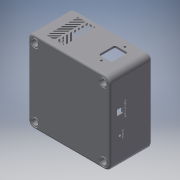
# Autodesk Inventor part: BottomBox
Saved by Autodesk Inventor 2019 (Build 230136000, 136)
## iProperties
Created: 2021-01-17
Part Number: BottomBox
Material: Типовые
Document SubType Name: Modeling
Designer: Dazer
Density: 1 g/cm^3
Appearance: По умолчанию
Author: Dazer
## iProperties of the stored document BottomBox_3DПЕЧАТЬ.ipt
Created: 2021-01-18
Part Number: BottomBox_3DПЕЧАТЬ
Material: Типовые
Document SubType Name: Modeling
Designer: Dazer
Density: 1 g/cm^3
Appearance: По умолчанию
Author: Dazer
Autodesk Inventor part; units mm, degrees
(part 1 of 2)
ref_plane "YZ Plane" through (0, 0, 0) normal (1, 0, 0) x (0, 1, 0)
ref_plane "XZ Plane" through (0, 0, 0) normal (0, 1, 0) x (-1, 0, 0)
ref_plane "XY Plane" through (0, 0, 0) normal (0, 0, 1) x (1, 0, 0)
sketch "Эскиз1" plane through (0, 0, 0) normal (0, 0, 1) x (1, 0, 0)
  circle A0 centre (1.5, -6.375) radius 2 projected
  circle A1 centre (88.9, -6.375) radius 2 projected
  circle A2 centre (88.9, -93.775) radius 2 projected
  circle A3 centre (1.5, -93.775) radius 2 projected
  arc A4 (87.4, -89.275) -> (84.4, -92.275) centre (87.4, -92.275) ccw projected
  line L0 (84.4, -92.275) -> (84.4, -96.775) projected
  arc A5 (81.4, -99.775) -> (84.4, -96.775) centre (81.4, -96.775) ccw projected
  line L1 (9, -99.775) -> (81.4, -99.775) projected
  arc A6 (6, -96.775) -> (9, -99.775) centre (9, -96.775) ccw projected
  line L2 (6, -96.775) -> (6, -92.275) projected
  arc A7 (6, -92.275) -> (3, -89.275) centre (3, -92.275) ccw projected
  line L3 (3, -89.275) -> (-1.5, -89.275) projected
  arc A8 (-4.5, -86.275) -> (-1.5, -89.275) centre (-1.5, -86.275) ccw projected
  line L4 (-4.5, -13.875) -> (-4.5, -86.275) projected
  arc A9 (-1.5, -10.875) -> (-4.5, -13.875) centre (-1.5, -13.875) ccw projected
  line L5 (-1.5, -10.875) -> (3, -10.875) projected
  arc A10 (3, -10.875) -> (6, -7.875) centre (3, -7.875) ccw projected
  line L6 (6, -7.875) -> (6, -3.375) projected
  arc A11 (9, -0.375) -> (6, -3.375) centre (9, -3.375) ccw projected
  line L7 (81.4, -0.375) -> (9, -0.375) projected
  arc A12 (84.4, -3.375) -> (81.4, -0.375) centre (81.4, -3.375) ccw projected
  line L8 (84.4, -3.375) -> (84.4, -7.875) projected
  arc A13 (84.4, -7.875) -> (87.4, -10.875) centre (87.4, -7.875) ccw projected
  line L9 (87.4, -10.875) -> (91.9, -10.875) projected
  arc A14 (94.9, -13.875) -> (91.9, -10.875) centre (91.9, -13.875) ccw projected
  line L10 (94.9, -86.275) -> (94.9, -13.875) projected
  arc A15 (91.9, -89.275) -> (94.9, -86.275) centre (91.9, -86.275) ccw projected
  line L11 (91.9, -89.275) -> (87.4, -89.275) projected
  line L12 (90.4, 0.875) -> (0, 0.875) projected
  arc A16 (0, 0.875) -> (-5.75, -4.875) centre (0, -4.875) ccw projected
  line L13 (-5.75, -4.875) -> (-5.75, -95.275) projected
  arc A17 (-5.75, -95.275) -> (0, -101.025) centre (0, -95.275) ccw projected
  line L14 (0, -101.025) -> (90.4, -101.025) projected
  arc A18 (90.4, -101.025) -> (96.15, -95.275) centre (90.4, -95.275) ccw projected
  line L15 (96.15, -95.275) -> (96.15, -4.875) projected
  arc A19 (96.15, -4.875) -> (90.4, 0.875) centre (90.4, -4.875) ccw projected
  line L16 (90.4, 0.775) -> (0, 0.775)
  arc A20 (0, 0.775) -> (-5.65, -4.875) centre (0, -4.875) ccw
  line L17 (-5.65, -4.875) -> (-5.65, -95.275)
  arc A21 (-5.65, -95.275) -> (0, -100.925) centre (0, -95.275) ccw
  line L18 (0, -100.925) -> (90.4, -100.925)
  arc A22 (90.4, -100.925) -> (96.05, -95.275) centre (90.4, -95.275) ccw
  line L19 (96.05, -95.275) -> (96.05, -4.875)
  arc A23 (96.05, -4.875) -> (90.4, 0.775) centre (90.4, -4.875) ccw
  circle A24 centre (88.9, -6.375) radius 2.3
  circle A25 centre (88.9, -93.775) radius 2.3
  circle A26 centre (1.5, -93.775) radius 2.3
  circle A27 centre (1.5, -6.375) radius 2.3
  point P0 (0, 0)
  dimension "d0" = 0.1
  dimension "d1" = 0.3
  dimension "d2" = 0.3
  dimension "d3" = 0.3
  dimension "d4" = 0.3
  constraints: 8 centre point, 8 end point, 8 point on circle, 7 other
  measures "d0" radial gap between concentric circles of A19 A23
  measures "d1" radial gap between concentric circles of A1 A24
  measures "d2" radial gap between concentric circles of A2 A25
  measures "d3" radial gap between concentric circles of A3 A26
  measures "d4" radial gap between concentric circles of A0 A27
extrude "Выдавливание1" add sketch "Эскиз1" along normal blind 2.1 contours A23 L19 A22 L18 A21 L17 A20 L16
sketch "Эскиз2" plane through (0, 0, 2.1) normal (0, 0, 1) x (1, 0, 0)
  arc A0 (96.15, -4.875) -> (90.4, 0.875) centre (90.4, -4.875) ccw projected
  line L0 (96.15, -4.875) -> (96.15, -95.275) projected
  arc A1 (90.4, -101.025) -> (96.15, -95.275) centre (90.4, -95.275) ccw projected
  line L1 (90.4, -101.025) -> (0, -101.025) projected
  arc A2 (-5.75, -95.275) -> (0, -101.025) centre (0, -95.275) ccw projected
  line L2 (-5.75, -95.275) -> (-5.75, -4.875) projected
  arc A3 (0, 0.875) -> (-5.75, -4.875) centre (0, -4.875) ccw projected
  line L3 (0, 0.875) -> (90.4, 0.875) projected
  line L4 (97.4, -95.275) -> (97.4, -4.875) projected
  arc A4 (97.4, -4.875) -> (90.4, 2.125) centre (90.4, -4.875) ccw projected
  line L5 (90.4, 2.125) -> (0, 2.125) projected
  arc A5 (0, 2.125) -> (-7, -4.875) centre (0, -4.875) ccw projected
  line L6 (-7, -4.875) -> (-7, -95.275) projected
  arc A6 (-7, -95.275) -> (0, -102.275) centre (0, -95.275) ccw projected
  line L7 (0, -102.275) -> (90.4, -102.275) projected
  arc A7 (90.4, -102.275) -> (97.4, -95.275) centre (90.4, -95.275) ccw projected
  line L8 (84.4, -92.275) -> (84.4, -96.775) projected
  arc A8 (81.4, -99.775) -> (84.4, -96.775) centre (81.4, -96.775) ccw projected
  line L9 (81.4, -99.775) -> (9, -99.775) projected
  arc A9 (6, -96.775) -> (9, -99.775) centre (9, -96.775) ccw projected
  line L10 (6, -96.775) -> (6, -92.275) projected
  arc A10 (6, -92.275) -> (3, -89.275) centre (3, -92.275) ccw projected
  line L11 (3, -89.275) -> (-1.5, -89.275) projected
  arc A11 (-4.5, -86.275) -> (-1.5, -89.275) centre (-1.5, -86.275) ccw projected
  line L12 (-4.5, -86.275) -> (-4.5, -13.875) projected
  arc A12 (-1.5, -10.875) -> (-4.5, -13.875) centre (-1.5, -13.875) ccw projected
  line L13 (-1.5, -10.875) -> (3, -10.875) projected
  arc A13 (3, -10.875) -> (6, -7.875) centre (3, -7.875) ccw projected
  line L14 (6, -7.875) -> (6, -3.375) projected
  arc A14 (9, -0.375) -> (6, -3.375) centre (9, -3.375) ccw projected
  line L15 (9, -0.375) -> (81.4, -0.375) projected
  arc A15 (84.4, -3.375) -> (81.4, -0.375) centre (81.4, -3.375) ccw projected
  line L16 (84.4, -3.375) -> (84.4, -7.875) projected
  arc A16 (84.4, -7.875) -> (87.4, -10.875) centre (87.4, -7.875) ccw projected
  line L17 (87.4, -10.875) -> (91.9, -10.875) projected
  arc A17 (94.9, -13.875) -> (91.9, -10.875) centre (91.9, -13.875) ccw projected
  line L18 (94.9, -13.875) -> (94.9, -86.275) projected
  arc A18 (91.9, -89.275) -> (94.9, -86.275) centre (91.9, -86.275) ccw projected
  line L19 (91.9, -89.275) -> (87.4, -89.275) projected
  arc A19 (87.4, -89.275) -> (84.4, -92.275) centre (87.4, -92.275) ccw projected
  circle A20 centre (1.5, -6.375) radius 2.3 projected
  circle A21 centre (1.5, -93.775) radius 2.3 projected
  circle A22 centre (88.9, -93.775) radius 2.3 projected
  circle A23 centre (88.9, -6.375) radius 2.3 projected
  line L20 (90.4, 0.775) -> (0, 0.775) projected
  arc A24 (0, 0.775) -> (-5.65, -4.875) centre (0, -4.875) ccw projected
  line L21 (-5.65, -4.875) -> (-5.65, -95.275) projected
  arc A25 (-5.65, -95.275) -> (0, -100.925) centre (0, -95.275) ccw projected
  line L22 (0, -100.925) -> (90.4, -100.925) projected
  arc A26 (90.4, -100.925) -> (96.05, -95.275) centre (90.4, -95.275) ccw projected
  line L23 (96.05, -95.275) -> (96.05, -4.875) projected
  arc A27 (96.05, -4.875) -> (90.4, 0.775) centre (90.4, -4.875) ccw projected
  point P0 (0, 0)
extrude "Выдавливание2" add sketch "Эскиз2" along normal blind 49 contours L0 A1 L1 A2 L2 A3 L3 A0 | A7 L7 A6 L6 A5 L5 A4 L4 | A27 L23 A26 L22 A25 L21 A24 L20
sketch "Эскиз3" plane through (0, 0, 51.1) normal (0, 0, 1) x (1, 0, 0)
  arc A0 (81.4, -99.775) -> (84.4, -96.775) centre (81.4, -96.775) ccw projected
  line L0 (81.4, -99.775) -> (9, -99.775) projected
  arc A1 (6, -96.775) -> (9, -99.775) centre (9, -96.775) ccw projected
  line L1 (6, -96.775) -> (6, -92.275) projected
  arc A2 (6, -92.275) -> (3, -89.275) centre (3, -92.275) ccw projected
  line L2 (3, -89.275) -> (-1.5, -89.275) projected
  arc A3 (-4.5, -86.275) -> (-1.5, -89.275) centre (-1.5, -86.275) ccw projected
  line L3 (-4.5, -86.275) -> (-4.5, -13.875) projected
  arc A4 (-1.5, -10.875) -> (-4.5, -13.875) centre (-1.5, -13.875) ccw projected
  line L4 (-1.5, -10.875) -> (3, -10.875) projected
  arc A5 (3, -10.875) -> (6, -7.875) centre (3, -7.875) ccw projected
  line L5 (6, -7.875) -> (6, -3.375) projected
  arc A6 (9, -0.375) -> (6, -3.375) centre (9, -3.375) ccw projected
  line L6 (9, -0.375) -> (81.4, -0.375) projected
  arc A7 (84.4, -3.375) -> (81.4, -0.375) centre (81.4, -3.375) ccw projected
  line L7 (84.4, -3.375) -> (84.4, -7.875) projected
  arc A8 (84.4, -7.875) -> (87.4, -10.875) centre (87.4, -7.875) ccw projected
  line L8 (87.4, -10.875) -> (91.9, -10.875) projected
  arc A9 (94.9, -13.875) -> (91.9, -10.875) centre (91.9, -13.875) ccw projected
  line L9 (94.9, -13.875) -> (94.9, -86.275) projected
  arc A10 (91.9, -89.275) -> (94.9, -86.275) centre (91.9, -86.275) ccw projected
  line L10 (91.9, -89.275) -> (87.4, -89.275) projected
  arc A11 (87.4, -89.275) -> (84.4, -92.275) centre (87.4, -92.275) ccw projected
  line L11 (84.4, -92.275) -> (84.4, -96.775) projected
  circle A12 centre (88.9, -6.375) radius 2.3 projected
  circle A13 centre (88.9, -93.775) radius 2.3 projected
  circle A14 centre (1.5, -93.775) radius 2.3 projected
  circle A15 centre (1.5, -6.375) radius 2.3 projected
  line L12 (97.4, -95.275) -> (97.4, -4.875) projected
  arc A16 (97.4, -4.875) -> (90.4, 2.125) centre (90.4, -4.875) ccw projected
  line L13 (90.4, 2.125) -> (0, 2.125) projected
  arc A17 (0, 2.125) -> (-7, -4.875) centre (0, -4.875) ccw projected
  line L14 (-7, -4.875) -> (-7, -95.275) projected
  arc A18 (-7, -95.275) -> (0, -102.275) centre (0, -95.275) ccw projected
  line L15 (0, -102.275) -> (90.4, -102.275) projected
  arc A19 (90.4, -102.275) -> (97.4, -95.275) centre (90.4, -95.275) ccw projected
  point P0 (0, 0)
extrude "Выдавливание3" add sketch "Эскиз3" along normal blind 2.5 contours L0 A1 L1 A2 L2 A3 L3 A4 L4 A5 L5 A6 L6 A7 L7 A8 L8 A9 L9 A10 L10 A11 L11 A0 | A19 L15 A18 L14 A17 L13 A16 L12
fillet "Сопряжение1" radius 2.5 8 edges at (-4.9497, -100.2247, 53.6) (45.2, -102.275, 53.6) (95.3497, -100.2247, 53.6) (97.4, -50.075, 53.6) (95.3497, 0.0747, 53.6) (45.2, 2.125, 53.6) (-4.9497, 0.0747, 53.6) (-7, -50.075, 53.6)
sketch "Эскиз5" plane through (0, 0, 53.6) normal (0, 0, 1) x (1, 0, 0)
  circle A0 centre (1.5, -6.375) radius 2.3 projected
  circle A1 centre (88.9, -6.375) radius 2.3 projected
  circle A2 centre (88.9, -93.775) radius 2.3 projected
  circle A3 centre (1.5, -93.775) radius 2.3 projected
  circle A4 centre (1.5, -93.775) radius 3.5
  circle A5 centre (88.9, -93.775) radius 3.5
  circle A6 centre (88.9, -6.375) radius 3.5
  circle A7 centre (1.5, -6.375) radius 3.5
  point P0 (0, 0)
  dimension "d22" = 7
  dimension "d23" = 7
  dimension "d24" = 7
  dimension "d25" = 7
  constraints: 4 centre point, 4 coincident
  measures "d22" diameter of A4
  measures "d23" diameter of A5
  measures "d24" diameter of A6
  measures "d25" diameter of A7
extrude "Выдавливание5" cut sketch "Эскиз5" against normal blind 39 contours A0 | A1 | A2 | A3 | A4 | A5 | A6 | A7
sketch "Эскиз6" plane through (97.4, -95.275, 2.1) normal (1, 0, 0) x (0, 0, -1)
  line L0 (-42.4, 54.65) -> (-42.4, 51.15)
  line L1 (-42.4, 58.15) -> (-42.4, 54.65)
  line L2 (-42.4, 58.15) -> (-34.78, 58.15)
  line L3 (-34.78, 58.15) -> (-34.78, 51.15)
  line L4 (-34.78, 51.15) -> (-42.4, 51.15)
  circle A0 centre (-38.59, 27.98) radius 1.5
  point P0 (2.1, 95.275)
  constraints: 10 end point, 1 centre point, 1 horizontal, 1 perpendicular, 1 point on line
extrude "Выдавливание6" cut sketch "Эскиз6" against normal blind 2.5
sketch "Эскиз7" plane through (0, 0, 51.1) normal (0, 0, -1) x (-1, 0, 0)
  arc A0 (-6, -7.875) -> (-3, -10.875) centre (-3, -7.875) ccw projected
  line L0 (-3, -89.275) -> (1.5, -89.275) projected
  line L1 (-3, -10.875) -> (-3, -89.275)
  line L2 (-3, -10.875) -> (1.5, -10.875)
  arc A1 (4.5, -13.875) -> (1.5, -10.875) centre (1.5, -13.875) ccw projected
  line L3 (4.5, -13.875) -> (4.5, -86.275)
  arc A2 (1.5, -89.275) -> (4.5, -86.275) centre (1.5, -86.275) ccw projected
  line L4 (-3, -89.275) -> (1.5, -89.275)
  arc A3 (1.5, -89.275) -> (4.5, -86.275) centre (1.5, -86.275) ccw
  arc A4 (4.5, -13.875) -> (1.5, -10.875) centre (1.5, -13.875) ccw
  point P0 (0, 0)
  constraints: 8 end point, 6 point on circle, 2 centre point, 2 tangent, 1 collinear, 1 concentric, 1 horizontal, 1 perpendicular, 1 vertical
extrude "Выдавливание7" add sketch "Эскиз7" along normal blind 5
sketch "Эскиз8" plane through (0, 0, 51.1) normal (0, 0, -1) x (-1, 0, 0)
  arc A0 (-6, -7.875) -> (-3, -10.875) centre (-3, -7.875) ccw projected
  line L0 (-6, -7.875) -> (-34, -7.875)
  line L1 (-34, -7.875) -> (-34, -0.375)
  line L2 (-34, -0.375) -> (-9, -0.375)
  arc A1 (-6, -3.375) -> (-9, -0.375) centre (-9, -3.375) ccw projected
  line L3 (-6, -3.375) -> (-6, -7.875)
  arc A2 (-6, -3.375) -> (-9, -0.375) centre (-9, -3.375) ccw
  line L4 (-6, -92.275) -> (-6, -96.775) projected
  line L5 (-6, -92.275) -> (-34, -92.275)
  line L6 (-34, -92.275) -> (-34, -99.775)
  line L7 (-81.4, -99.775) -> (-9, -99.775) projected
  arc A3 (-9, -99.775) -> (-6, -96.775) centre (-9, -96.775) ccw projected
  line L8 (-34, -99.775) -> (-9, -99.775)
  arc A4 (-3, -89.275) -> (-6, -92.275) centre (-3, -92.275) ccw projected
  line L9 (-6, -92.275) -> (-6, -96.775)
  arc A5 (-9, -99.775) -> (-6, -96.775) centre (-9, -96.775) ccw
  arc A6 (-84.4, -92.275) -> (-87.4, -89.275) centre (-87.4, -92.275) ccw projected
  line L10 (-84.4, -92.275) -> (-74.4, -92.275)
  line L11 (-74.4, -92.275) -> (-74.4, -99.775)
  line L12 (-9, -99.775) -> (-81.4, -99.775) projected
  line L13 (-74.4, -99.775) -> (-81.4, -99.775)
  arc A7 (-84.4, -96.775) -> (-81.4, -99.775) centre (-81.4, -96.775) ccw projected
  line L14 (-84.4, -92.275) -> (-84.4, -96.775)
  arc A8 (-84.4, -96.775) -> (-81.4, -99.775) centre (-81.4, -96.775) ccw
  line L15 (-64.4, -0.375) -> (-64.4, -7.375)
  line L16 (-64.4, -7.375) -> (-69.4, -7.375)
  line L17 (-69.4, -7.375) -> (-69.4, -0.375)
  line L18 (-69.4, -0.375) -> (-64.4, -0.375)
  point P0 (0, 0)
  dimension "d43" = 28
  dimension "d46" = 28
  dimension "d47" = 10
  constraints: 32 end point, 8 point on circle, 7 tangent, 6 horizontal, 4 perpendicular, 4 vertical, 3 centre point, 2 point on line, 1 concentric
  measures "d43" distance of L0.start L0.end
  measures "d46" distance of L4.start L5.end
  measures "d47" distance of L10.start L10.end
extrude "Выдавливание8" add sketch "Эскиз8" along normal blind 5
fillet "Сопряжение2" radius 2.5 5 edges at (34, -7.875, 48.6) (34, -92.275, 48.6) (74.4, -92.275, 48.6) (64.4, -7.375, 48.6) (69.4, -7.375, 48.6)
fillet "Сопряжение3" radius 2.5 12 edges at (49.2, -0.375, 51.1) (85.2787, -9.9963, 51.1) (89.65, -10.875, 51.1) (94.0213, -11.7537, 51.1) (94.9, -50.075, 51.1) (94.0213, -88.3963, 51.1) (89.65, -89.275, 51.1) (85.2787, -90.1537, 51.1) (83.5213, -1.2537, 51.1) (75.4, -0.375, 51.1) (84.4, -5.625, 51.1) (54.2, -99.775, 51.1)
fillet "Сопряжение4" radius 2.5 2 edges at (5.1213, -90.1537, 51.1) (5.1213, -9.9963, 51.1)
sketch "Эскиз9" plane through (0, 2.125, 2.1) normal (0, 1, 0) x (1, 0, 0)
  line L0 (9, -4) -> (11.5, -4)
  line L1 (9, -4) -> (9, -6.5)
  line L2 (9, -6.5) -> (11.5, -4)
  line L3 (9, -14) -> (19, -4)
  line L4 (9, -14) -> (9, -16.5)
  line L5 (9, -19) -> (9, -21.5)
  line L6 (9, -34) -> (9, -36.5)
  line L7 (9, -39) -> (9, -41.5)
  line L8 (19, -4) -> (19, -6.5)
  line L9 (19, -9) -> (19, -11.5)
  line L10 (19, -24) -> (19, -26.5)
  line L11 (19, -29) -> (19, -31.5)
  line L12 (9, -16.5) -> (19, -6.5)
  line L13 (9, -19) -> (19, -9)
  line L14 (9, -21.5) -> (19, -11.5)
  line L15 (9, -24) -> (19, -14)
  line L16 (9, -26.5) -> (19, -16.5)
  line L17 (9, -29) -> (19, -19)
  line L18 (9, -31.5) -> (19, -21.5)
  line L19 (9, -34) -> (19, -24)
  line L20 (9, -36.5) -> (19, -26.5)
  line L21 (9, -39) -> (19, -29)
  line L22 (9, -41.5) -> (19, -31.5)
  line L23 (9, -44) -> (19, -34)
  line L24 (11.5, -44) -> (19, -36.5)
  line L25 (14, -44) -> (19, -39)
  line L26 (16.5, -44) -> (19, -41.5)
  line L27 (9, -9) -> (14, -4)
  line L28 (9, -11.5) -> (16.5, -4)
  line L29 (14, -4) -> (16.5, -4)
  line L30 (9, -9) -> (9, -11.5)
  line L31 (19, -34) -> (19, -36.5)
  line L32 (11.5, -44) -> (9, -44)
  line L33 (14, -44) -> (16.5, -44)
  line L34 (19, -39) -> (19, -41.5)
  line L35 (9, -24) -> (9, -26.5)
  line L36 (19, -14) -> (19, -16.5)
  line L37 (9, -29) -> (9, -31.5)
  line L38 (19, -21.5) -> (19, -19)
  line L39 (31.5, -4) -> (29, -4)
  line L40 (31.5, -4) -> (31.5, -6.5)
  line L41 (31.5, -6.5) -> (29, -4)
  line L42 (31.5, -14) -> (21.5, -4)
  line L43 (31.5, -14) -> (31.5, -16.5)
  line L44 (31.5, -19) -> (31.5, -21.5)
  line L45 (31.5, -34) -> (31.5, -36.5)
  line L46 (31.5, -39) -> (31.5, -41.5)
  line L47 (21.5, -4) -> (21.5, -6.5)
  line L48 (21.5, -9) -> (21.5, -11.5)
  line L49 (21.5, -24) -> (21.5, -26.5)
  line L50 (21.5, -29) -> (21.5, -31.5)
  line L51 (31.5, -16.5) -> (21.5, -6.5)
  line L52 (31.5, -19) -> (21.5, -9)
  line L53 (31.5, -21.5) -> (21.5, -11.5)
  line L54 (31.5, -24) -> (21.5, -14)
  line L55 (31.5, -26.5) -> (21.5, -16.5)
  line L56 (31.5, -29) -> (21.5, -19)
  line L57 (31.5, -31.5) -> (21.5, -21.5)
  line L58 (31.5, -34) -> (21.5, -24)
  line L59 (31.5, -36.5) -> (21.5, -26.5)
  line L60 (31.5, -39) -> (21.5, -29)
  line L61 (31.5, -41.5) -> (21.5, -31.5)
  line L62 (31.5, -44) -> (21.5, -34)
  line L63 (29, -44) -> (21.5, -36.5)
  line L64 (26.5, -44) -> (21.5, -39)
  line L65 (24, -44) -> (21.5, -41.5)
  line L66 (31.5, -9) -> (26.5, -4)
  line L67 (31.5, -11.5) -> (24, -4)
  line L68 (26.5, -4) -> (24, -4)
  line L69 (31.5, -9) -> (31.5, -11.5)
  line L70 (21.5, -34) -> (21.5, -36.5)
  line L71 (29, -44) -> (31.5, -44)
  line L72 (26.5, -44) -> (24, -44)
  line L73 (21.5, -39) -> (21.5, -41.5)
  line L74 (31.5, -24) -> (31.5, -26.5)
  line L75 (21.5, -14) -> (21.5, -16.5)
  line L76 (31.5, -29) -> (31.5, -31.5)
  line L77 (21.5, -21.5) -> (21.5, -19)
  point P0 (0, 2.1)
  constraints: 156 end point, 16 parallel, 4 point on line, 2 perpendicular, 2 vertical, 1 collinear, 1 horizontal
extrude "Выдавливание9" cut sketch "Эскиз9" against normal blind 120
sketch "Эскиз10" plane through (0, -102.275, 2.1) normal (0, -1, 0) x (1, 0, 0)
  line L0 (31.5, 19) -> (21.5, 9) projected
  line L1 (21.5, 9) -> (21.5, 11.5) projected
  line L2 (21.5, 11.5) -> (31.5, 21.5) projected
  line L3 (31.5, 21.5) -> (31.5, 19) projected
  line L4 (31.5, 31.5) -> (31.5, 29) projected
  line L5 (31.5, 29) -> (21.5, 19) projected
  line L6 (21.5, 19) -> (21.5, 21.5) projected
  line L7 (21.5, 21.5) -> (31.5, 31.5) projected
  line L8 (31.5, 39) -> (21.5, 29) projected
  line L9 (21.5, 29) -> (21.5, 31.5) projected
  line L10 (21.5, 31.5) -> (31.5, 41.5) projected
  line L11 (31.5, 41.5) -> (31.5, 39) projected
  line L12 (9, 21.5) -> (19, 11.5) projected
  line L13 (19, 11.5) -> (19, 9) projected
  line L14 (19, 9) -> (9, 19) projected
  line L15 (9, 19) -> (9, 21.5) projected
  line L16 (9, 29) -> (9, 31.5) projected
  line L17 (9, 31.5) -> (19, 21.5) projected
  line L18 (19, 21.5) -> (19, 19) projected
  line L19 (19, 19) -> (9, 29) projected
  line L20 (9, 41.5) -> (19, 31.5) projected
  line L21 (19, 31.5) -> (19, 29) projected
  line L22 (19, 29) -> (9, 39) projected
  line L23 (9, 39) -> (9, 41.5) projected
  line L24 (9, 44) -> (11.5, 44) projected
  line L25 (11.5, 44) -> (19, 36.5) projected
  line L26 (19, 36.5) -> (19, 34) projected
  line L27 (19, 34) -> (9, 44) projected
  line L28 (9, 9) -> (9, 11.5) projected
  line L29 (9, 11.5) -> (16.5, 4) projected
  line L30 (16.5, 4) -> (14, 4) projected
  line L31 (14, 4) -> (9, 9) projected
  line L32 (14, 44) -> (16.5, 44) projected
  line L33 (16.5, 44) -> (19, 41.5) projected
  line L34 (19, 41.5) -> (19, 39) projected
  line L35 (19, 39) -> (14, 44) projected
  line L36 (9, 4) -> (9, 6.5) projected
  line L37 (9, 6.5) -> (11.5, 4) projected
  line L38 (11.5, 4) -> (9, 4) projected
  line L39 (31.5, 4) -> (29, 4) projected
  line L40 (29, 4) -> (31.5, 6.5) projected
  line L41 (31.5, 6.5) -> (31.5, 4) projected
  line L42 (21.5, 39) -> (21.5, 41.5) projected
  line L43 (21.5, 41.5) -> (24, 44) projected
  line L44 (24, 44) -> (26.5, 44) projected
  line L45 (26.5, 44) -> (21.5, 39) projected
  line L46 (26.5, 4) -> (24, 4) projected
  line L47 (24, 4) -> (31.5, 11.5) projected
  line L48 (31.5, 11.5) -> (31.5, 9) projected
  line L49 (31.5, 9) -> (26.5, 4) projected
  line L50 (21.5, 34) -> (21.5, 36.5) projected
  line L51 (21.5, 36.5) -> (29, 44) projected
  line L52 (29, 44) -> (31.5, 44) projected
  line L53 (31.5, 44) -> (21.5, 34) projected
  line L54 (9, 36.5) -> (19, 26.5) projected
  line L55 (19, 26.5) -> (19, 24) projected
  line L56 (19, 24) -> (9, 34) projected
  line L57 (9, 34) -> (9, 36.5) projected
  line L58 (9, 24) -> (9, 26.5) projected
  line L59 (9, 26.5) -> (19, 16.5) projected
  line L60 (19, 16.5) -> (19, 14) projected
  line L61 (19, 14) -> (9, 24) projected
  line L62 (9, 14) -> (9, 16.5) projected
  line L63 (9, 16.5) -> (19, 6.5) projected
  line L64 (19, 6.5) -> (19, 4) projected
  line L65 (19, 4) -> (9, 14) projected
  line L66 (21.5, 26.5) -> (31.5, 36.5) projected
  line L67 (31.5, 36.5) -> (31.5, 34) projected
  line L68 (31.5, 34) -> (21.5, 24) projected
  line L69 (21.5, 24) -> (21.5, 26.5) projected
  line L70 (21.5, 14) -> (21.5, 16.5) projected
  line L71 (21.5, 16.5) -> (31.5, 26.5) projected
  line L72 (31.5, 26.5) -> (31.5, 24) projected
  line L73 (31.5, 24) -> (21.5, 14) projected
  line L74 (21.5, 4) -> (21.5, 6.5) projected
  line L75 (21.5, 6.5) -> (31.5, 16.5) projected
  line L76 (31.5, 16.5) -> (31.5, 14) projected
  line L77 (31.5, 14) -> (21.5, 4) projected
  line L78 (0, 49) -> (90.4, 49) projected
  line L79 (0, 0) -> (0, 49) projected
  line L80 (0, 0) -> (90.4, 0) projected
  line L81 (90.4, 0) -> (90.4, 49) projected
  line L82 (31.5, 31.5) -> (31.5, 29) projected
  line L83 (45.2, 4) -> (45.2, 22.7)
  line L84 (58.9, 19) -> (68.9, 9)
  line L85 (68.9, 9) -> (68.9, 11.5)
  line L86 (68.9, 11.5) -> (58.9, 21.5)
  line L87 (58.9, 21.5) -> (58.9, 19)
  line L88 (58.9, 31.5) -> (58.9, 29)
  line L89 (58.9, 29) -> (68.9, 19)
  line L90 (68.9, 19) -> (68.9, 21.5)
  line L91 (68.9, 21.5) -> (58.9, 31.5)
  line L92 (58.9, 39) -> (68.9, 29)
  line L93 (68.9, 29) -> (68.9, 31.5)
  line L94 (68.9, 31.5) -> (58.9, 41.5)
  line L95 (58.9, 41.5) -> (58.9, 39)
  line L96 (81.4, 21.5) -> (71.4, 11.5)
  line L97 (71.4, 11.5) -> (71.4, 9)
  line L98 (71.4, 9) -> (81.4, 19)
  line L99 (81.4, 19) -> (81.4, 21.5)
  line L100 (81.4, 29) -> (81.4, 31.5)
  line L101 (81.4, 31.5) -> (71.4, 21.5)
  line L102 (71.4, 21.5) -> (71.4, 19)
  line L103 (71.4, 19) -> (81.4, 29)
  line L104 (81.4, 41.5) -> (71.4, 31.5)
  line L105 (71.4, 31.5) -> (71.4, 29)
  line L106 (71.4, 29) -> (81.4, 39)
  line L107 (81.4, 39) -> (81.4, 41.5)
  line L108 (81.4, 44) -> (78.9, 44)
  line L109 (78.9, 44) -> (71.4, 36.5)
  line L110 (71.4, 36.5) -> (71.4, 34)
  line L111 (71.4, 34) -> (81.4, 44)
  line L112 (81.4, 9) -> (81.4, 11.5)
  line L113 (81.4, 11.5) -> (73.9, 4)
  line L114 (73.9, 4) -> (76.4, 4)
  line L115 (76.4, 4) -> (81.4, 9)
  line L116 (76.4, 44) -> (73.9, 44)
  line L117 (73.9, 44) -> (71.4, 41.5)
  line L118 (71.4, 41.5) -> (71.4, 39)
  line L119 (71.4, 39) -> (76.4, 44)
  line L120 (81.4, 4) -> (81.4, 6.5)
  line L121 (81.4, 6.5) -> (78.9, 4)
  line L122 (78.9, 4) -> (81.4, 4)
  line L123 (58.9, 4) -> (61.4, 4)
  line L124 (61.4, 4) -> (58.9, 6.5)
  line L125 (58.9, 6.5) -> (58.9, 4)
  line L126 (68.9, 39) -> (68.9, 41.5)
  line L127 (68.9, 41.5) -> (66.4, 44)
  line L128 (66.4, 44) -> (63.9, 44)
  line L129 (63.9, 44) -> (68.9, 39)
  line L130 (63.9, 4) -> (66.4, 4)
  line L131 (66.4, 4) -> (58.9, 11.5)
  line L132 (58.9, 11.5) -> (58.9, 9)
  line L133 (58.9, 9) -> (63.9, 4)
  line L134 (68.9, 34) -> (68.9, 36.5)
  line L135 (68.9, 36.5) -> (61.4, 44)
  line L136 (61.4, 44) -> (58.9, 44)
  line L137 (58.9, 44) -> (68.9, 34)
  line L138 (81.4, 36.5) -> (71.4, 26.5)
  line L139 (71.4, 26.5) -> (71.4, 24)
  line L140 (71.4, 24) -> (81.4, 34)
  line L141 (81.4, 34) -> (81.4, 36.5)
  line L142 (81.4, 24) -> (81.4, 26.5)
  line L143 (81.4, 26.5) -> (71.4, 16.5)
  line L144 (71.4, 16.5) -> (71.4, 14)
  line L145 (71.4, 14) -> (81.4, 24)
  line L146 (81.4, 14) -> (81.4, 16.5)
  line L147 (81.4, 16.5) -> (71.4, 6.5)
  line L148 (71.4, 6.5) -> (71.4, 4)
  line L149 (71.4, 4) -> (81.4, 14)
  line L150 (68.9, 26.5) -> (58.9, 36.5)
  line L151 (58.9, 36.5) -> (58.9, 34)
  line L152 (58.9, 34) -> (68.9, 24)
  line L153 (68.9, 24) -> (68.9, 26.5)
  line L154 (68.9, 14) -> (68.9, 16.5)
  line L155 (68.9, 16.5) -> (58.9, 26.5)
  line L156 (58.9, 26.5) -> (58.9, 24)
  line L157 (58.9, 24) -> (68.9, 14)
  line L158 (68.9, 4) -> (68.9, 6.5)
  line L159 (68.9, 6.5) -> (58.9, 16.5)
  line L160 (58.9, 16.5) -> (58.9, 14)
  line L161 (58.9, 14) -> (68.9, 4)
  line L162 (58.9, 31.5) -> (58.9, 29)
  constraints: 160 end point, 78 symmetric about line, 1 vertical
extrude "Выдавливание10" cut sketch "Эскиз10" against normal blind 2.5 contours L87 L86 L85 L84 | L91 L90 L89 L88 | L95 L94 L93 L92 | L99 L98 L97 L96 | L103 L102 L101 L100 | L107 L106 L105 L104 | L111 L110 L109 L108 | L115 L114 L113 L112 | L119 L118 L117 L116 | L122 L121 L120 | L125 L124 L123 | L129 L128 L127 L126 | L133 L132 L131 L130 | L137 L136 L135 L134 | L141 L140 L139 L138 | L145 L144 L143 L142 | L149 L148 L147 L146 | L153 L152 L151 L150 | L157 L156 L155 L154 | L161 L160 L159 L158
sketch "Эскиз11" plane through (-7, -95.275, 2.1) normal (-1, 0, 0) x (0, 0, 1)
  circle A0 centre (8.95, 54.4) radius 1.5
  circle A1 centre (8.95, 78.4) radius 1.5
  circle A2 centre (32.95, 54.4) radius 1.5
  circle A3 centre (32.95, 78.4) radius 1.5
  line L0 (11.45, 51.4) -> (13.45, 51.4)
  line L1 (15.95, 51.4) -> (18.45, 51.4)
  line L2 (25.95, 51.4) -> (28.45, 51.4)
  line L3 (28.45, 81.4) -> (25.95, 81.4)
  line L4 (5.95, 73.9) -> (5.95, 71.4)
  line L5 (5.95, 63.9) -> (5.95, 61.4)
  line L6 (5.95, 58.9) -> (5.95, 56.9)
  line L7 (13.45, 51.4) -> (11.6085, 53.2415)
  line L8 (15.95, 51.4) -> (11.4028, 55.9472)
  line L9 (18.45, 51.4) -> (5.95, 63.9)
  line L10 (10.4972, 56.8528) -> (5.95, 61.4)
  line L11 (7.7915, 57.0585) -> (5.95, 58.9)
  line L12 (20.95, 51.4) -> (5.95, 66.4)
  line L13 (23.45, 51.4) -> (5.95, 68.9)
  line L14 (25.95, 51.4) -> (5.95, 71.4)
  line L15 (28.45, 51.4) -> (5.95, 73.9)
  line L16 (30.45, 51.9) -> (6.45, 75.9)
  line L17 (30.0744, 54.7756) -> (9.3256, 75.5244)
  line L18 (30.8994, 56.4506) -> (10.95, 76.4)
  line L19 (32.5744, 57.2756) -> (11.8256, 78.0244)
  line L20 (35.45, 56.9) -> (11.45, 80.9)
  line L21 (35.95, 58.9) -> (13.45, 81.4)
  line L22 (35.95, 61.4) -> (15.95, 81.4)
  line L23 (18.45, 81.4) -> (35.95, 63.9)
  line L24 (35.95, 66.4) -> (20.95, 81.4)
  line L25 (35.95, 68.9) -> (23.45, 81.4)
  line L26 (35.95, 71.4) -> (31.4028, 75.9472)
  line L27 (30.4972, 76.8528) -> (25.95, 81.4)
  line L28 (30.2915, 79.5585) -> (28.45, 81.4)
  line L29 (35.95, 73.9) -> (34.1085, 75.7415)
  line L30 (20.95, 51.4) -> (23.45, 51.4)
  line L31 (5.95, 66.4) -> (5.95, 68.9)
  line L32 (11.45, 81.4) -> (13.45, 81.4)
  line L33 (15.95, 81.4) -> (18.45, 81.4)
  line L34 (20.95, 81.4) -> (23.45, 81.4)
  line L35 (35.95, 56.9) -> (35.95, 58.9)
  line L36 (35.95, 61.4) -> (35.95, 63.9)
  line L37 (35.95, 66.4) -> (35.95, 68.9)
  line L38 (35.95, 71.4) -> (35.95, 73.9)
  line L39 (21.7965, 45.2) -> (45.6778, 45.2)
  line L40 (7.4803, 75.9) -> (6.45, 75.9)
  line L41 (11.45, 80.9) -> (11.45, 81.4)
  line L42 (11.45, 52.9303) -> (11.45, 51.4)
  line L43 (7.4803, 56.9) -> (5.95, 56.9)
  line L44 (30.45, 52.9303) -> (30.45, 51.9)
  line L45 (35.45, 56.9) -> (35.95, 56.9)
  circle A4 centre (8.95, 36) radius 1.5
  circle A5 centre (8.95, 12) radius 1.5
  circle A6 centre (32.95, 36) radius 1.5
  circle A7 centre (32.95, 12) radius 1.5
  line L46 (11.45, 39) -> (13.45, 39)
  line L47 (15.95, 39) -> (18.45, 39)
  line L48 (25.95, 39) -> (28.45, 39)
  line L49 (28.45, 9) -> (25.95, 9)
  line L50 (5.95, 16.5) -> (5.95, 19)
  line L51 (5.95, 26.5) -> (5.95, 29)
  line L52 (5.95, 31.5) -> (5.95, 33.5)
  line L53 (13.45, 39) -> (11.6085, 37.1585)
  line L54 (15.95, 39) -> (11.4028, 34.4528)
  line L55 (18.45, 39) -> (5.95, 26.5)
  line L56 (10.4972, 33.5472) -> (5.95, 29)
  line L57 (7.7915, 33.3415) -> (5.95, 31.5)
  line L58 (20.95, 39) -> (5.95, 24)
  line L59 (23.45, 39) -> (5.95, 21.5)
  line L60 (25.95, 39) -> (5.95, 19)
  line L61 (28.45, 39) -> (5.95, 16.5)
  line L62 (30.45, 38.5) -> (6.45, 14.5)
  line L63 (30.0744, 35.6244) -> (9.3256, 14.8756)
  line L64 (30.8994, 33.9494) -> (11.0006, 14.0506)
  line L65 (32.5744, 33.1244) -> (11.8256, 12.3756)
  line L66 (35.45, 33.5) -> (11.45, 9.5)
  line L67 (35.95, 31.5) -> (13.45, 9)
  line L68 (35.95, 29) -> (15.95, 9)
  line L69 (18.45, 9) -> (35.95, 26.5)
  line L70 (35.95, 24) -> (20.95, 9)
  line L71 (35.95, 21.5) -> (23.45, 9)
  line L72 (35.95, 19) -> (31.4028, 14.4528)
  line L73 (30.4972, 13.5472) -> (25.95, 9)
  line L74 (30.2915, 10.8415) -> (28.45, 9)
  line L75 (35.95, 16.5) -> (34.1085, 14.6585)
  line L76 (20.95, 39) -> (23.45, 39)
  line L77 (5.95, 24) -> (5.95, 21.5)
  line L78 (11.45, 9) -> (13.45, 9)
  line L79 (15.95, 9) -> (18.45, 9)
  line L80 (20.95, 9) -> (23.45, 9)
  line L81 (35.95, 33.5) -> (35.95, 31.5)
  line L82 (35.95, 29) -> (35.95, 26.5)
  line L83 (35.95, 24) -> (35.95, 21.5)
  line L84 (35.95, 19) -> (35.95, 16.5)
  line L85 (7.4803, 14.5) -> (6.45, 14.5)
  line L86 (11.45, 9.5) -> (11.45, 9)
  line L87 (11.45, 37.4697) -> (11.45, 39)
  line L88 (7.4803, 33.5) -> (5.95, 33.5)
  line L89 (30.45, 37.4697) -> (30.45, 38.5)
  line L90 (35.45, 33.5) -> (35.95, 33.5)
  arc A8 (7.4803, 33.5) -> (7.7915, 33.3415) centre (8.95, 36) ccw
  arc A9 (10.4972, 33.5472) -> (11.4028, 34.4528) centre (8.95, 36) ccw
  arc A10 (11.6085, 37.1585) -> (11.45, 37.4697) centre (8.95, 36) ccw
  arc A11 (34.1085, 14.6585) -> (31.4028, 14.4528) centre (32.95, 12) ccw
  arc A12 (30.4972, 13.5472) -> (30.2915, 10.8415) centre (32.95, 12) ccw
  arc A13 (11.8256, 12.3756) -> (11.0006, 14.0506) centre (8.95, 12) ccw
  arc A14 (9.3256, 14.8756) -> (7.4803, 14.5) centre (8.95, 12) ccw
  arc A15 (30.45, 37.4697) -> (30.0744, 35.6244) centre (32.95, 36) ccw
  arc A16 (30.8994, 33.9494) -> (32.5744, 33.1244) centre (32.95, 36) ccw
  arc A17 (30.2915, 79.5585) -> (30.4972, 76.8528) centre (32.95, 78.4) ccw
  arc A18 (31.4028, 75.9472) -> (34.1085, 75.7415) centre (32.95, 78.4) ccw
  arc A19 (32.5744, 57.2756) -> (30.8994, 56.4506) centre (32.95, 54.4) ccw
  arc A20 (30.0744, 54.7756) -> (30.45, 52.9303) centre (32.95, 54.4) ccw
  arc A21 (11.0006, 76.3494) -> (11.8256, 78.0244) centre (8.95, 78.4) ccw
  arc A22 (7.4803, 75.9) -> (9.3256, 75.5244) centre (8.95, 78.4) ccw
  arc A23 (11.45, 52.9303) -> (11.6085, 53.2415) centre (8.95, 54.4) ccw
  arc A24 (11.4028, 55.9472) -> (10.4972, 56.8528) centre (8.95, 54.4) ccw
  arc A25 (7.7915, 57.0585) -> (7.4803, 56.9) centre (8.95, 54.4) ccw
  point P0 (-2.1, 95.275)
  constraints: 182 end point, 42 symmetric about line, 36 point on circle, 26 centre point, 16 parallel, 5 perpendicular, 5 point on line, 3 collinear, 3 horizontal, 3 vertical, 1 coincident, 4 other
extrude "Выдавливание12" cut sketch "Эскиз11" against normal blind 2.5
sketch "Эскиз13" plane through (-7, -95.275, 2.1) normal (-1, 0, 0) x (0, 0, 1)
  circle A0 centre (8.95, 12) radius 1.5 projected
  circle A1 centre (8.95, 36) radius 1.5 projected
  circle A2 centre (32.95, 12) radius 1.5 projected
  circle A3 centre (32.95, 36) radius 1.5 projected
  circle A4 centre (32.95, 54.4) radius 1.5 projected
  circle A5 centre (8.95, 54.4) radius 1.5 projected
  circle A6 centre (8.95, 78.4) radius 1.5 projected
  circle A7 centre (32.95, 78.4) radius 1.5 projected
  point P0 (-2.1, 95.275)
hole "Отверстие1" at (-7, -83.275, 11.05) at (-7, -83.275, 35.05) at (-7, -59.275, 35.05) at (-7, -59.275, 11.05) at (-7, -40.875, 11.05) at (-7, -40.875, 35.05) at (-7, -16.875, 35.05) at (-7, -16.875, 11.05) direction (1, 0, 0) diameter 3 depth 8 tip angle 118 countersink diameter 5.8 countersink angle 90
sketch "Эскиз15" plane through (0, 2.125, 2.1) normal (0, 1, 0) x (1, 0, 0)
  line L0 (90.4, 2.1) -> (0, 2.1) projected
  circle A0 centre (72.05, -6.95) radius 1.35
  circle A1 centre (72.05, -36.95) radius 1.35
  line L1 (80.4, -13.5698) -> (80.4, -30.5)
  line L2 (78.5501, -32.3499) -> (65.8, -32.3499)
  line L3 (78.4, -11.5698) -> (65.8, -11.5698)
  line L4 (63.8, -13.5698) -> (63.8, -30.3499)
  line L5 (78.5501, -32.3499) -> (78.4, -32.3499)
  arc A2 (63.8, -30.3499) -> (65.8, -32.3499) centre (65.8, -30.3499) ccw
  arc A3 (78.2499, -32.3499) -> (80.4, -30.1999) centre (78.4, -30.3499) ccw
  arc A4 (65.8, -11.5698) -> (63.8, -13.5698) centre (65.8, -13.5698) ccw
  arc A5 (80.4, -13.5698) -> (78.4, -11.5698) centre (78.4, -13.5698) ccw
  point P0 (81.4, 2.1)
  point P1 (64.4, -44)
  constraints: 10 end point, 10 point on circle, 6 centre point, 4 point on line, 3 tangent, 2 perpendicular, 1 horizontal, 1 vertical
extrude "Выдавливание13" cut sketch "Эскиз15" against normal blind 2.5 contours A0 | A1 | L1 A3 L2 A2 L4 A4 L3 A5
sketch "Эскиз16" plane through (-7, -95.275, 2.1) normal (-1, 0, 0) x (0, 0, 1)
  arc A0 (7.4803, 14.5) -> (11.8256, 12.3756) centre (8.95, 12) ccw projected
  circle A1 centre (8.95, 12) radius 1.5 projected
  arc A2 (11.4028, 34.4528) -> (11.6085, 37.1585) centre (8.95, 36) ccw projected
  circle A3 centre (8.95, 36) radius 1.5 projected
  arc A4 (32.5744, 33.1244) -> (30.45, 37.4697) centre (32.95, 36) ccw projected
  circle A5 centre (32.95, 36) radius 1.5 projected
  arc A6 (30.2915, 10.8415) -> (34.1085, 14.6585) centre (32.95, 12) ccw projected
  circle A7 centre (32.95, 12) radius 1.5 projected
  arc A8 (30.45, 52.9303) -> (32.5744, 57.2756) centre (32.95, 54.4) ccw projected
  circle A9 centre (32.95, 54.4) radius 1.5 projected
  arc A10 (34.1085, 75.7415) -> (30.2915, 79.5585) centre (32.95, 78.4) ccw projected
  circle A11 centre (32.95, 78.4) radius 1.5 projected
  arc A12 (11.8256, 78.0244) -> (7.4803, 75.9) centre (8.95, 78.4) ccw projected
  circle A13 centre (8.95, 78.4) radius 1.5 projected
  arc A14 (11.6085, 53.2415) -> (11.4028, 55.9472) centre (8.95, 54.4) ccw projected
  circle A15 centre (8.95, 54.4) radius 1.5 projected
  arc A16 (8.95, 15.4) -> (12.35, 12) centre (8.95, 12) ccw
  arc A17 (11.75, 13.8) -> (8.95, 15.4) centre (9.0949, 12.4035) ccw
  arc A18 (12.35, 12) -> (11.75, 13.8) centre (9.35, 12) ccw
  circle A19 centre (8.95, 36) radius 3.4
  circle A20 centre (8.95, 54.4) radius 3.4
  arc A21 (12.35, 78.4) -> (8.95, 75) centre (8.95, 78.4) ccw
  arc A22 (11.35, 76.2) -> (12.35, 78.4) centre (9.3502, 78.4363) ccw
  arc A23 (8.95, 75) -> (11.35, 76.2) centre (8.95, 78) ccw
  arc A24 (32.95, 75) -> (29.55, 78.4) centre (32.95, 78.4) ccw
  arc A25 (30.75, 76) -> (32.95, 75) centre (32.9863, 77.9998) ccw
  arc A26 (30.15, 76.6) -> (30.75, 76) centre (32.55, 78.4) ccw
  arc A27 (29.55, 78.4) -> (30.15, 76.6) centre (32.55, 78.4) ccw
  arc A28 (29.55, 54.4) -> (32.95, 57.8) centre (32.95, 54.4) ccw
  arc A29 (31.15, 57.2) -> (29.55, 54.4) centre (32.5465, 54.5449) ccw
  arc A30 (32.95, 57.8) -> (31.15, 57.2) centre (32.95, 54.8) ccw
  arc A31 (32.95, 32.6) -> (29.55, 36) centre (32.95, 36) ccw
  arc A32 (30.75, 33.6) -> (32.95, 32.6) centre (32.9863, 35.5998) ccw
  arc A33 (29.55, 36) -> (30.75, 33.6) centre (32.55, 36) ccw
  arc A34 (29.95, 12) -> (32.95, 15) centre (32.95, 12) ccw
  arc A35 (32.95, 15) -> (31.15, 14.4) centre (32.95, 12) ccw
  arc A36 (31.15, 14.4) -> (30.55, 13.8) centre (32.95, 12) ccw
  arc A37 (30.55, 13.8) -> (29.95, 12) centre (32.95, 12) ccw
  arc A38 (11.4028, 55.9472) -> (10.4972, 56.8528) centre (8.95, 54.4) ccw projected
  arc A39 (10.4972, 56.8528) -> (7.7915, 57.0585) centre (8.95, 54.4) ccw projected
  arc A40 (7.7915, 57.0585) -> (7.4803, 56.9) centre (8.95, 54.4) ccw projected
  arc A41 (7.4803, 56.9) -> (11.45, 52.9303) centre (8.95, 54.4) ccw projected
  arc A42 (11.45, 52.9303) -> (11.6085, 53.2415) centre (8.95, 54.4) ccw projected
  arc A43 (7.4803, 75.9) -> (9.3256, 75.5244) centre (8.95, 78.4) ccw projected
  arc A44 (9.3256, 75.5244) -> (11.0006, 76.3494) centre (8.95, 78.4) ccw projected
  arc A45 (11.0006, 76.3494) -> (11.8256, 78.0244) centre (8.95, 78.4) ccw projected
  arc A46 (30.2915, 79.5585) -> (30.4972, 76.8528) centre (32.95, 78.4) ccw projected
  arc A47 (30.4972, 76.8528) -> (31.4028, 75.9472) centre (32.95, 78.4) ccw projected
  arc A48 (31.4028, 75.9472) -> (34.1085, 75.7415) centre (32.95, 78.4) ccw projected
  arc A49 (32.5744, 57.2756) -> (30.8994, 56.4506) centre (32.95, 54.4) ccw projected
  arc A50 (30.8994, 56.4506) -> (30.0744, 54.7756) centre (32.95, 54.4) ccw projected
  arc A51 (30.0744, 54.7756) -> (30.45, 52.9303) centre (32.95, 54.4) ccw projected
  arc A52 (34.1085, 14.6585) -> (31.4028, 14.4528) centre (32.95, 12) ccw projected
  arc A53 (31.4028, 14.4528) -> (30.4972, 13.5472) centre (32.95, 12) ccw projected
  arc A54 (30.4972, 13.5472) -> (30.2915, 10.8415) centre (32.95, 12) ccw projected
  arc A55 (30.45, 37.4697) -> (30.0744, 35.6244) centre (32.95, 36) ccw projected
  arc A56 (30.0744, 35.6244) -> (30.8994, 33.9494) centre (32.95, 36) ccw projected
  arc A57 (30.8994, 33.9494) -> (32.5744, 33.1244) centre (32.95, 36) ccw projected
  arc A58 (11.6085, 37.1585) -> (11.45, 37.4697) centre (8.95, 36) ccw projected
  arc A59 (11.45, 37.4697) -> (7.4803, 33.5) centre (8.95, 36) ccw projected
  arc A60 (7.4803, 33.5) -> (7.7915, 33.3415) centre (8.95, 36) ccw projected
  arc A61 (7.7915, 33.3415) -> (10.4972, 33.5472) centre (8.95, 36) ccw projected
  arc A62 (10.4972, 33.5472) -> (11.4028, 34.4528) centre (8.95, 36) ccw projected
  arc A63 (11.8256, 12.3756) -> (11.0006, 14.0506) centre (8.95, 12) ccw projected
  arc A64 (11.0006, 14.0506) -> (9.3256, 14.8756) centre (8.95, 12) ccw projected
  arc A65 (9.3256, 14.8756) -> (7.4803, 14.5) centre (8.95, 12) ccw projected
  point P0 (-2.1, 95.275)
  dimension "d228" = 0.5
  dimension "d229" = 0.5
  dimension "d230" = 0.5
  dimension "d231" = 0.5
  dimension "d232" = 0.5
  dimension "d233" = 0.5
  dimension "d234" = 0.5
  constraints: 40 point on circle, 22 centre point
  measures "d228" radial gap between concentric circles of A0 A16
  measures "d229" radial gap between concentric circles of A2 A19
  measures "d230" radial gap between concentric circles of A14 A20
  measures "d231" radial gap between concentric circles of A12 A21
  measures "d232" radial gap between concentric circles of A10 A24
  measures "d233" radial gap between concentric circles of A8 A28
  measures "d234" radial gap between concentric circles of A4 A31
extrude "Выдавливание14" add sketch "Эскиз16" against normal blind 2.5 contours A17 A18 A16 | A19 | A20 | A22 A23 A21 | A25 A26 A27 A24 | A29 A30 A28 | A32 A33 A31 | A37 A36 A35 A34